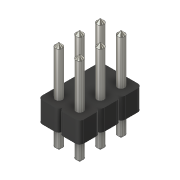
# Autodesk Inventor part: 2x3 header
Saved by Autodesk Inventor 2020 (Build 240168000, 168)
## iProperties
Created: 2017-10-26
Part Number: 2x3 header
Material: Generic
Document SubType Name: Modeling
Designer: Alex
Density: 1 g/cm^3
Appearance: Default
Author: Alex
Autodesk Inventor part; units mm, degrees
ref_plane "YZ Plane" through (0, 0, 0) normal (1, 0, 0) x (0, 1, 0)
ref_plane "XZ Plane" through (0, 0, 0) normal (0, 1, 0) x (-1, 0, 0)
ref_plane "XY Plane" through (0, 0, 0) normal (0, 0, 1) x (1, 0, 0)
sketch "Sketch1" plane through (0, 0, 0) normal (0, 1, 0) x (-1, 0, 0)
  line L0 (-1.778, 6.35) -> (-3.302, 6.35)
  arc A0 (-3.302, 6.35) -> (-3.81, 5.842) centre (-3.302, 5.842) ccw
  line L1 (-3.81, 5.842) -> (-3.81, 4.318)
  arc A1 (-3.81, 4.318) -> (-3.302, 3.81) centre (-3.302, 4.318) ccw
  arc A2 (-3.302, 3.81) -> (-3.81, 3.302) centre (-3.302, 3.302) ccw
  line L2 (-3.81, 3.302) -> (-3.81, 1.778)
  arc A3 (-3.81, 1.778) -> (-3.302, 1.27) centre (-3.302, 1.778) ccw
  arc A4 (-3.302, 1.27) -> (-3.81, 0.762) centre (-3.302, 0.762) ccw
  line L3 (-3.81, 0.762) -> (-3.81, -0.762)
  arc A5 (-3.81, -0.762) -> (-3.302, -1.27) centre (-3.302, -0.762) ccw
  line L4 (-3.302, -1.27) -> (-1.778, -1.27)
  arc A6 (-1.778, -1.27) -> (-1.27, -0.762) centre (-1.778, -0.762) ccw
  arc A7 (-1.27, -0.762) -> (-0.762, -1.27) centre (-0.762, -0.762) ccw
  line L5 (-0.762, -1.27) -> (0.762, -1.27)
  arc A8 (0.762, -1.27) -> (1.27, -0.762) centre (0.762, -0.762) ccw
  line L6 (1.27, -0.762) -> (1.27, 0.762)
  arc A9 (1.27, 0.762) -> (0.762, 1.27) centre (0.762, 0.762) ccw
  arc A10 (0.762, 1.27) -> (1.27, 1.778) centre (0.762, 1.778) ccw
  line L7 (1.27, 1.778) -> (1.27, 3.302)
  arc A11 (1.27, 3.302) -> (0.762, 3.81) centre (0.762, 3.302) ccw
  arc A12 (0.762, 3.81) -> (1.27, 4.318) centre (0.762, 4.318) ccw
  line L8 (1.27, 4.318) -> (1.27, 5.842)
  arc A13 (1.27, 5.842) -> (0.762, 6.35) centre (0.762, 5.842) ccw
  line L9 (0.762, 6.35) -> (-0.762, 6.35)
  arc A14 (-0.762, 6.35) -> (-1.27, 5.842) centre (-0.762, 5.842) ccw
  arc A15 (-1.27, 5.842) -> (-1.778, 6.35) centre (-1.778, 5.842) ccw
  arc A16 (-1.27, 0.762) -> (-1.778, 1.27) centre (-1.778, 0.762) ccw
  arc A17 (-1.778, 1.27) -> (-1.27, 1.778) centre (-1.778, 1.778) ccw
  arc A18 (-1.27, 1.778) -> (-0.762, 1.27) centre (-0.762, 1.778) ccw
  arc A19 (-0.762, 1.27) -> (-1.27, 0.762) centre (-0.762, 0.762) ccw
  arc A20 (-1.27, 3.302) -> (-1.778, 3.81) centre (-1.778, 3.302) ccw
  arc A21 (-1.778, 3.81) -> (-1.27, 4.318) centre (-1.778, 4.318) ccw
  arc A22 (-1.27, 4.318) -> (-0.762, 3.81) centre (-0.762, 4.318) ccw
  arc A23 (-0.762, 3.81) -> (-1.27, 3.302) centre (-0.762, 3.302) ccw
  constraints: 48 point on circle, 24 centre point, 20 end point
extrude "Extrusion1" add sketch "Sketch1" along normal blind 2.54
sketch "Sketch2" plane through (0, 2.54, 0) normal (0, 1, 0) x (1, 0, 0)
  circle A0 centre (0, 0) radius 0.4445
  line L0 (0.762, 1.27) -> (-0.762, 1.27) construction
  line L1 (-1.27, 0.762) -> (-1.27, -0.762) construction
  circle A1 centre (2.54, 0) radius 0.4445
  circle A2 centre (0, -2.54) radius 0.4445
  circle A3 centre (2.54, -2.54) radius 0.4445
  circle A4 centre (0, -5.08) radius 0.4445
  circle A5 centre (2.54, -5.08) radius 0.4445
  dimension "d2" = 0.889
  dimension "d5" = 2.54
  dimension "d8" = 2.54
  constraints: 6 centre point, 6 coincident, 1 horizontal, 1 vertical, 15 other
  measures "d2" diameter of A0
  measures "d5" distance of point (0, 0) point (2.54, 0)
  measures "d8" distance of point (0, 0) point (0, -2.54)
extrude "Extrusion2" add sketch "Sketch2" along normal blind 5.842 and the other way blind 5.4356
chamfer "Chamfer1" distance 0.381 angle 45 12 edges at (2.0955, 8.382, 5.08) (-0.4445, 8.382, 5.08) (2.0955, 8.382, 2.54) (-0.4445, 8.382, 2.54) (2.0955, 8.382, 0) (-0.4445, 8.382, 0) (2.0955, -2.8956, 5.08) (2.0955, -2.8956, 2.54) (2.0955, -2.8956, 0) (-0.4445, -2.8956, 0) (-0.4445, -2.8956, 2.54) (-0.4445, -2.8956, 5.08)
body "Solid1"
